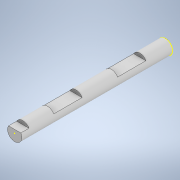
# Autodesk Inventor part: 3SR03_振子軸
Saved by Autodesk Inventor 2021 (Build 250183000, 183)
## iProperties
Created: 2021-04-20
Part Number: 3SR03_振子軸
Material: 一般
Document SubType Name: Modeling
Designer: ryusei
Density: 1 g/cm^3
Appearance: 既定
Author: ryusei
Autodesk Inventor part; units mm, degrees
ref_plane "YZ Plane" through (0, 0, 0) normal (1, 0, 0) x (0, 1, 0)
ref_plane "XZ Plane" through (0, 0, 0) normal (0, 1, 0) x (-1, 0, 0)
ref_plane "XY Plane" through (0, 0, 0) normal (0, 0, 1) x (1, 0, 0)
sketch "スケッチ1" plane through (0, 0, 0) normal (0, 0, 1) x (1, 0, 0)
  circle A0 centre (0, 0) radius 2
  dimension "d0" = 4
  constraints: 1 centre point, 1 coincident
  measures "d0" diameter of A0
extrude "押し出し1" add sketch "スケッチ1" along normal blind 42.5
sketch "スケッチ2" plane through (0, 0, 42.5) normal (0, 0, 1) x (1, 0, 0)
  circle A0 centre (0, 0) radius 2 projected
  line L0 (-1.7321, 1) -> (1.7321, 1)
  dimension "d3" = 1
  constraints: 2 end point, 2 point on circle, 1 horizontal
  measures "d3" distance centre to line of A0 L0
extrude "押し出し2" cut sketch "スケッチ2" against normal blind 2.3 contours L0 A0 picked at (0.4849, 1.1242)
sketch "スケッチ3" plane through (0, 0, 42.5) normal (0, 0, 1) x (1, 0, 0)
  point P0 (0, 0)
sketch "スケッチ4" plane through (0, 0, 0) normal (0, 0, -1) x (-1, 0, 0)
  arc A0 (1.7321, 1) -> (-1.7321, 1) centre (0, 0) ccw projected
  circle A1 centre (0, 0) radius 2 projected
sketch "スケッチ5" plane through (-1.7321, 1, 42.5) normal (0, 1, 0) x (1, 0, 0)
  point P0 (1.7321, 42.5)
sketch "スケッチ6" plane through (-1.7321, 1, 42.5) normal (0, 1, 0) x (1, 0, 0)
  line L0 (-15.0722, 17.3) -> (4.9278, 17.3)
  line L1 (4.9278, 17.3) -> (4.9278, 9.3)
  line L2 (4.9278, 9.3) -> (-15.0722, 9.3)
  line L3 (-15.0722, 9.3) -> (-15.0722, 17.3)
  line L4 (3.4641, 2.3) -> (0, 2.3) projected
  line L5 (-8.306, 35.3) -> (11.694, 35.3)
  line L6 (11.694, 35.3) -> (11.694, 27.3)
  line L7 (11.694, 27.3) -> (-8.306, 27.3)
  line L8 (-8.306, 27.3) -> (-8.306, 35.3)
  point P0 (1.7321, 42.5)
  dimension "d8" = 8
  dimension "d9" = 20
  dimension "d10" = 15
  dimension "d12" = 20
  dimension "d13" = 25
  dimension "d16" = 8
  constraints: 16 end point, 4 parallel, 2 horizontal, 2 perpendicular
  measures "d8" distance between parallel lines of L2 L0
  measures "d9" distance between parallel lines of L1 L3
  measures "d10" distance between parallel lines of L4 L0
  measures "d12" distance between parallel lines of L6 L8
  measures "d13" distance between parallel lines of L7 L4
  measures "d16" distance between parallel lines of L7 L5
extrude "押し出し3" cut sketch "スケッチ6" along normal blind 10
